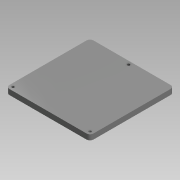
# Autodesk Inventor part: Print Bed
Saved by Autodesk Inventor 2016 (Build 200138000, 138)
## iProperties
Created: 2017-05-15
Part Number: Print Bed
Material: Generic
Document SubType Name: Modeling
Designer: 31745
Density: 1 g/cm^3
Appearance: Default
Author: 31745
Autodesk Inventor part; units mm, degrees
ref_plane "YZ Plane" through (0, 0, 0) normal (1, 0, 0) x (0, 1, 0)
ref_plane "XZ Plane" through (0, 0, 0) normal (0, 1, 0) x (-1, 0, 0)
ref_plane "XY Plane" through (0, 0, 0) normal (0, 0, 1) x (1, 0, 0)
sketch "Sketch1" plane through (0, 0, 0) normal (0, 1, 0) x (-1, 0, 0)
  line L0 (0, 0) -> (-152.4, 0)
  line L1 (-152.4, 0) -> (-152.4, -152.4)
  line L2 (-152.4, -152.4) -> (0, -152.4)
  line L3 (0, -152.4) -> (0, 0)
  dimension "d0" = 152.4
  dimension "d1" = 152.4
  constraints: 8 end point, 2 parallel, 1 horizontal, 1 perpendicular
  measures "d0" distance of L0.start L0.end
  measures "d1" distance of L2.end L0.start
extrude "Extrusion1" add sketch "Sketch1" along normal blind 9.525
fillet "Fillet1" radius 6.35 4 edges at (152.4, 4.7625, 0) (152.4, 4.7625, -152.4) (0, 4.7625, -152.4) (0, 4.7625, 0)
sketch "Sketch3" plane through (0, 9.525, 0) normal (0, 1, 0) x (1, 0, 0)
  arc A0 (0, 6.35) -> (6.35, 0) centre (6.35, 6.35) ccw projected
  line L0 (6.35, 0) -> (146.05, 0) projected
  arc A1 (146.05, 0) -> (152.4, 6.35) centre (146.05, 6.35) ccw projected
  line L1 (152.4, 6.35) -> (152.4, 146.05) projected
  arc A2 (152.4, 146.05) -> (146.05, 152.4) centre (146.05, 146.05) ccw projected
  line L2 (146.05, 152.4) -> (6.35, 152.4) projected
  arc A3 (6.35, 152.4) -> (0, 146.05) centre (6.35, 146.05) ccw projected
  line L3 (0, 146.05) -> (0, 6.35) projected
  point P0 (0, 0)
  point P1 (76.2, 146.05)
  point P2 (76.2, 152.4)
  constraints: 2 coincident, 1 horizontal alignment, 1 midpoint, 1 vertical alignment
hole "Hole1" at (6.35, 9.525, -6.35) at (146.05, 9.525, -6.35) at (76.2, 9.525, -146.05) direction (0, -1, 0) diameter 4.4958 end through all clearance for "Flat Head Machine Screw (82)" size "#8" standard "Ansi Unified Screw Threads"
body "Solid1"
